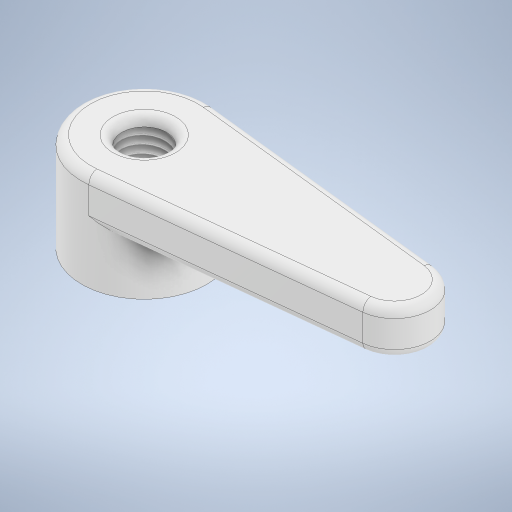
# Autodesk Inventor part: rapoukServoLegv0
Saved by Autodesk Inventor 2024 (Build 280153000, 153)
## iProperties
Created: 2024-01-30
Part Number: rapoukServoLegv0
Material: ABS Plastic
Document SubType Name: Modeling
Designer: S21Suk
Density: 1.06 g/cm^3
Appearance: Smooth - White
MASSSFP: 400 g
SFP: 4HR
Author: S21Suk
Autodesk Inventor part; units mm, degrees
ref_plane "YZ Plane" through (0, 0, 0) normal (1, 0, 0) x (0, 1, 0)
ref_plane "XZ Plane" through (0, 0, 0) normal (0, 1, 0) x (-1, 0, 0)
ref_plane "XY Plane" through (0, 0, 0) normal (0, 0, 1) x (1, 0, 0)
sketch "Náčrt2" plane through (0, 0, 0) normal (0, 1, 0) x (-1, 0, 0)
  arc A0 (-0.375, -3.4799) -> (-0.375, 3.4799) centre (0, 0) ccw
  circle A1 centre (0, 0) radius 1.25
  line L0 (0, 0) -> (-14, 0) construction
  arc A2 (-14.2143, 1.9885) -> (-14.2143, -1.9885) centre (-14, 0) ccw
  line L1 (-14.2143, 1.9885) -> (-0.375, 3.4799)
  line L2 (-14.2143, -1.9885) -> (-0.375, -3.4799)
  dimension "d2" = 7
  dimension "d3" = 2.5
  dimension "d4" = 14
  dimension "d5" = 4
  constraints: 6 end point, 4 point on circle, 4 tangent, 3 centre point, 3 coincident, 1 horizontal
  measures "d2" diameter of A0
  measures "d3" diameter of A1
  measures "d4" distance of L0.start L0.end
  measures "d5" diameter of A2
extrude "Vysunutí2" add sketch "Náčrt2" along normal blind 2.5
sketch "Náčrt3" plane through (0, 0, 0) normal (0, -1, 0) x (1, 0, 0)
  circle A0 centre (0, 0) radius 3.5
  circle A1 centre (0, 0) radius 1.5
  dimension "d8" = 7
  dimension "d9" = 3
  constraints: 2 centre point, 2 coincident
  measures "d8" diameter of A0
  measures "d9" diameter of A1
extrude "Vysunutí3" add sketch "Náčrt3" along normal blind 3
fillet "Zaoblení1" radius 0.5 8 edges at (-3.5, 2.5, 0) (7.2946, 2.5, 2.7342) (16, 2.5, 0) (7.2946, 2.5, -2.7342) (1.25, 2.5, 0) (16, 0, 0) (7.2946, 0, 2.7342) (7.2946, 0, -2.7342)
thread "Thread1" size "M2.5x0.45" class "6H" standard "ANSI Metric M Profile" full length
chamfer "Chamfer1" distance 0.2 angle 45 1 edges at (1.25, 0, 0)
